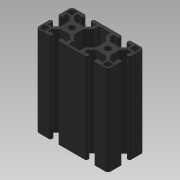
# Autodesk Inventor part: 40-4080-LITE-BLACK-FB
Saved by Autodesk Inventor 2013 (Build 170138000, 138)
## iProperties
Company: 80/20 Inc.
Created: 2014-04-23
Part Number: 40-4080-LITE-BLACK-FB
Material: Generic
Document SubType Name: Modeling
Designer: Ross Bowman
Density: 1 g/cm^3
Engineer: Ross Bowman
Catalog Web Link: 8020.net
Vendor: 80/20 Inc.
Material: 6105-T5 Aluminum
Author: Ross Bowman
Keywords: 80/20 , 8020 , T-Slot , Extrusion
Autodesk Inventor part; units mm, degrees
ref_plane "YZ Plane" through (0, 0, 0) normal (1, 0, 0) x (0, 1, 0)
ref_plane "XZ Plane" through (0, 0, 0) normal (0, 1, 0) x (-1, 0, 0)
ref_plane "XY Plane" through (0, 0, 0) normal (0, 0, 1) x (1, 0, 0)
sketch "Sketch1" plane through (0, 0, 0) normal (0, 0, 1) x (1, 0, 0)
  line L0 (31.935, -13.21) -> (31.935, -17.72)
  arc A0 (33.21, -11.94) -> (31.935, -13.21) centre (33.205, -13.21) ccw
  line L1 (37.72, -11.94) -> (33.21, -11.94)
  arc A1 (38.345, -12.57) -> (37.72, -11.94) centre (37.715, -12.57) ccw
  line L2 (38.345, -15.55) -> (38.345, -12.57)
  arc A2 (35.545, -18.35) -> (38.345, -15.55) centre (35.545, -15.55) ccw
  line L3 (32.565, -18.35) -> (35.545, -18.35)
  arc A3 (31.935, -17.72) -> (32.565, -18.35) centre (32.565, -17.72) ccw
  circle A4 centre (20, 0) radius 3.4
  line L4 (38.345, 12.57) -> (38.345, 15.55)
  arc A5 (37.72, 11.94) -> (38.345, 12.57) centre (37.715, 12.57) ccw
  line L5 (33.21, 11.94) -> (37.72, 11.94)
  arc A6 (31.935, 13.21) -> (33.21, 11.94) centre (33.205, 13.21) ccw
  line L6 (31.935, 17.72) -> (31.935, 13.21)
  arc A7 (32.565, 18.35) -> (31.935, 17.72) centre (32.565, 17.72) ccw
  line L7 (35.545, 18.35) -> (32.565, 18.35)
  arc A8 (38.345, 15.55) -> (35.545, 18.35) centre (35.545, 15.55) ccw
  line L8 (-38.345, -12.57) -> (-38.345, -15.55)
  arc A9 (-37.72, -11.94) -> (-38.345, -12.57) centre (-37.715, -12.57) ccw
  line L9 (-33.21, -11.94) -> (-37.72, -11.94)
  arc A10 (-31.935, -13.21) -> (-33.21, -11.94) centre (-33.205, -13.21) ccw
  line L10 (-31.935, -17.72) -> (-31.935, -13.21)
  arc A11 (-32.565, -18.35) -> (-31.935, -17.72) centre (-32.565, -17.72) ccw
  line L11 (-35.545, -18.35) -> (-32.565, -18.35)
  arc A12 (-38.345, -15.55) -> (-35.545, -18.35) centre (-35.545, -15.55) ccw
  line L12 (-10.9397, -6.7352) -> (-6.8324, -10.8426)
  arc A13 (-12.3289, -3.3756) -> (-10.9397, -6.7352) centre (-7.5789, -3.3786) ccw
  line L13 (-12.3247, 3.3825) -> (-12.3289, -3.3756)
  arc A14 (-10.9313, 6.7404) -> (-12.3247, 3.3825) centre (-7.5747, 3.3795) ccw
  line L14 (-6.8214, 10.8451) -> (-10.9313, 6.7404)
  arc A15 (-6.8214, 10.8451) -> (-6.4494, 11.7432) centre (-7.7194, 11.7432) ccw
  line L15 (-6.4494, 15.43) -> (-6.4494, 11.7432)
  arc A16 (-5.1787, 16.7) -> (-6.4494, 15.43) centre (-5.1794, 15.43) ccw
  line L16 (0, 16.6968) -> (-5.1787, 16.7)
  line L17 (5.1794, 16.7) -> (0, 16.6968)
  arc A17 (6.4494, 15.43) -> (5.1794, 16.7) centre (5.1794, 15.43) ccw
  line L18 (6.4494, 11.7432) -> (6.4494, 15.43)
  arc A18 (6.4494, 11.7432) -> (6.8214, 10.8451) centre (7.7194, 11.7432) ccw
  line L19 (10.9313, 6.7404) -> (6.8214, 10.8451)
  arc A19 (12.3247, 3.3825) -> (10.9313, 6.7404) centre (7.5747, 3.3795) ccw
  line L20 (12.3289, -3.3756) -> (12.3247, 3.3825)
  arc A20 (10.9376, -6.7373) -> (12.3289, -3.3756) centre (7.5789, -3.3786) ccw
  line L21 (6.8324, -10.8426) -> (10.9376, -6.7373)
  arc A21 (6.8324, -10.8426) -> (6.4604, -11.7406) centre (7.7304, -11.7406) ccw
  line L22 (6.4604, -16.4474) -> (6.4604, -11.7406)
  arc A22 (5.1904, -17.7174) -> (6.4604, -16.4474) centre (5.1904, -16.4474) ccw
  line L23 (-5.1904, -17.7174) -> (5.1904, -17.7174)
  arc A23 (-6.4604, -16.4474) -> (-5.1904, -17.7174) centre (-5.1904, -16.4474) ccw
  line L24 (-6.4604, -11.7406) -> (-6.4604, -16.4474)
  arc A24 (-6.4604, -11.7406) -> (-6.8324, -10.8426) centre (-7.7304, -11.7406) ccw
  circle A25 centre (-20, 0) radius 3.4
  line L25 (-37.72, 11.94) -> (-33.21, 11.94)
  arc A26 (-38.345, 12.57) -> (-37.72, 11.94) centre (-37.715, 12.57) ccw
  line L26 (-38.345, 15.55) -> (-38.345, 12.57)
  arc A27 (-35.545, 18.35) -> (-38.345, 15.55) centre (-35.545, 15.55) ccw
  line L27 (-32.565, 18.35) -> (-35.545, 18.35)
  arc A28 (-31.935, 17.72) -> (-32.565, 18.35) centre (-32.565, 17.72) ccw
  line L28 (-31.935, 13.21) -> (-31.935, 17.72)
  arc A29 (-33.21, 11.94) -> (-31.935, 13.21) centre (-33.205, 13.21) ccw
  arc A30 (-14.38, 20) -> (-15.94, 18.6069) centre (-14.38, 18.43) ccw
  line L29 (-15.94, 18.6069) -> (-15.94, 17.51)
  arc A31 (-15.94, 17.51) -> (-14.37, 15.94) centre (-14.37, 17.51) ccw
  line L30 (-14.37, 15.94) -> (-13.1517, 15.94)
  line L31 (-13.1517, 15.94) -> (-13.1517, 16.4117)
  line L32 (-13.1517, 16.4117) -> (-11.0437, 16.4117)
  arc A32 (-9.715, 15.1431) -> (-11.0437, 16.4117) centre (-10.985, 15.1431) ccw
  line L33 (-9.715, 15.1431) -> (-9.715, 12.8476)
  arc A33 (-9.9761, 12.2179) -> (-9.715, 12.8476) centre (-10.605, 12.8476) ccw
  line L34 (-9.9761, 12.2179) -> (-13.4586, 8.7397)
  arc A34 (-16.4245, 7.7) -> (-13.4586, 8.7397) centre (-16.4245, 12.45) ccw
  line L35 (-16.4245, 7.7) -> (-23.1872, 7.7)
  arc A35 (-26.7456, 9.087) -> (-23.1872, 7.7) centre (-23.3868, 12.4458) ccw
  line L36 (-26.7456, 9.087) -> (-30.0243, 12.3658)
  arc A36 (-30.285, 12.9951) -> (-30.0243, 12.3658) centre (-29.395, 12.9951) ccw
  line L37 (-30.285, 12.9951) -> (-30.285, 15.0869)
  arc A37 (-29.015, 16.3569) -> (-30.285, 15.0869) centre (-29.015, 15.0869) ccw
  line L38 (-29.015, 16.3569) -> (-26.8483, 16.3569)
  line L39 (-26.8483, 16.3569) -> (-26.8483, 15.8852)
  line L40 (-26.8483, 15.8852) -> (-25.63, 15.8852)
  arc A38 (-25.63, 15.8852) -> (-24.06, 17.4552) centre (-25.63, 17.4552) ccw
  line L41 (-24.06, 17.4552) -> (-24.06, 18.43)
  arc A39 (-24.06, 18.43) -> (-25.63, 20) centre (-25.63, 18.43) ccw
  line L42 (-25.63, 20) -> (-36.83, 20)
  arc A40 (-36.83, 20) -> (-40, 16.83) centre (-36.83, 16.83) ccw
  line L43 (-40, 16.83) -> (-40, 5.5719)
  arc A41 (-40, 5.5719) -> (-38.4311, 4.06) centre (-38.4311, 5.63) ccw
  line L44 (-38.4311, 4.06) -> (-37.51, 4.06)
  arc A42 (-37.51, 4.06) -> (-35.94, 5.63) centre (-37.51, 5.63) ccw
  line L45 (-35.94, 5.63) -> (-35.94, 6.6964)
  line L46 (-35.94, 6.6964) -> (-36.715, 6.6964)
  line L47 (-36.715, 6.6964) -> (-36.715, 9.02)
  arc A43 (-35.445, 10.29) -> (-36.715, 9.02) centre (-35.445, 9.02) ccw
  line L48 (-35.445, 10.29) -> (-33.1501, 10.29)
  arc A44 (-32.5208, 10.0293) -> (-33.1501, 10.29) centre (-33.1501, 9.4) ccw
  line L49 (-32.5208, 10.0293) -> (-29.0912, 6.5998)
  arc A45 (-27.7, 3.241) -> (-29.0912, 6.5998) centre (-32.45, 3.241) ccw
  line L50 (-27.7, 3.241) -> (-27.7, -3.241)
  arc A46 (-29.0912, -6.5998) -> (-27.7, -3.241) centre (-32.45, -3.241) ccw
  line L51 (-29.0912, -6.5998) -> (-32.5208, -10.0293)
  arc A47 (-33.1501, -10.29) -> (-32.5208, -10.0293) centre (-33.1501, -9.4) ccw
  line L52 (-33.1501, -10.29) -> (-35.445, -10.29)
  arc A48 (-36.715, -9.02) -> (-35.445, -10.29) centre (-35.445, -9.02) ccw
  line L53 (-36.715, -9.02) -> (-36.715, -6.6964)
  line L54 (-36.715, -6.6964) -> (-35.94, -6.6964)
  line L55 (-35.94, -6.6964) -> (-35.94, -5.63)
  arc A49 (-35.94, -5.63) -> (-37.51, -4.06) centre (-37.51, -5.63) ccw
  line L56 (-37.51, -4.06) -> (-38.4311, -4.06)
  arc A50 (-38.4311, -4.06) -> (-40, -5.5719) centre (-38.4311, -5.63) ccw
  line L57 (-40, -5.5719) -> (-40, -16.83)
  arc A51 (-40, -16.83) -> (-36.83, -20) centre (-36.83, -16.83) ccw
  line L58 (-36.83, -20) -> (-25.6944, -20)
  arc A52 (-25.6944, -20) -> (-24.06, -18.3656) centre (-25.6944, -18.3656) ccw
  line L59 (-24.06, -18.3656) -> (-24.06, -17.4474)
  arc A53 (-24.06, -17.4474) -> (-25.6944, -15.813) centre (-25.6944, -17.4474) ccw
  line L60 (-25.6944, -15.813) -> (-26.8283, -15.813)
  line L61 (-26.8283, -15.813) -> (-26.8283, -16.5584)
  line L62 (-26.8283, -16.5584) -> (-29.015, -16.5584)
  arc A54 (-30.285, -15.2884) -> (-29.015, -16.5584) centre (-29.015, -15.2884) ccw
  line L63 (-30.285, -15.2884) -> (-30.285, -12.8291)
  arc A55 (-30.0243, -12.1998) -> (-30.285, -12.8291) centre (-29.395, -12.8291) ccw
  line L64 (-30.0243, -12.1998) -> (-26.7392, -8.9146)
  arc A56 (-23.3804, -7.5234) -> (-26.7392, -8.9146) centre (-23.3804, -12.2734) ccw
  line L65 (-23.3804, -7.5234) -> (-16.6196, -7.5234)
  arc A57 (-13.2608, -8.9146) -> (-16.6196, -7.5234) centre (-16.6196, -12.2734) ccw
  line L66 (-13.2608, -8.9146) -> (-9.9757, -12.1998)
  arc A58 (-9.715, -12.8291) -> (-9.9757, -12.1998) centre (-10.605, -12.8291) ccw
  line L67 (-9.715, -12.8291) -> (-9.715, -15.3686)
  arc A59 (-11.0293, -16.5584) -> (-9.715, -15.3686) centre (-10.9825, -15.2892) ccw
  line L68 (-11.0293, -16.5584) -> (-13.1717, -16.5584)
  line L69 (-13.1717, -16.5584) -> (-13.1717, -15.813)
  line L70 (-13.1717, -15.813) -> (-14.3056, -15.813)
  arc A60 (-14.3056, -15.813) -> (-15.94, -17.4474) centre (-14.3056, -17.4474) ccw
  line L71 (-15.94, -17.4474) -> (-15.94, -18.3656)
  arc A61 (-15.94, -18.3656) -> (-14.3056, -20) centre (-14.3056, -18.3656) ccw
  line L72 (-14.3056, -20) -> (14.3056, -20)
  arc A62 (14.3056, -20) -> (15.94, -18.3656) centre (14.3056, -18.3656) ccw
  line L73 (15.94, -18.3656) -> (15.94, -17.4474)
  arc A63 (15.94, -17.4474) -> (14.3056, -15.813) centre (14.3056, -17.4474) ccw
  line L74 (14.3056, -15.813) -> (13.1717, -15.813)
  line L75 (13.1717, -15.813) -> (13.1717, -16.5584)
  line L76 (13.1717, -16.5584) -> (11.0293, -16.5584)
  arc A64 (9.715, -15.3686) -> (11.0293, -16.5584) centre (10.9825, -15.2892) ccw
  line L77 (9.715, -15.3686) -> (9.715, -12.8291)
  arc A65 (9.9757, -12.1998) -> (9.715, -12.8291) centre (10.605, -12.8291) ccw
  line L78 (9.9757, -12.1998) -> (13.2608, -8.9146)
  arc A66 (16.6196, -7.5234) -> (13.2608, -8.9146) centre (16.6196, -12.2734) ccw
  line L79 (16.6196, -7.5234) -> (23.3834, -7.5234)
  arc A67 (26.7392, -8.9146) -> (23.3834, -7.5234) centre (23.3804, -12.2734) ccw
  line L80 (26.7392, -8.9146) -> (30.0243, -12.1998)
  arc A68 (30.285, -12.8291) -> (30.0243, -12.1998) centre (29.395, -12.8291) ccw
  line L81 (30.285, -12.8291) -> (30.285, -15.2884)
  arc A69 (29.015, -16.5584) -> (30.285, -15.2884) centre (29.015, -15.2884) ccw
  line L82 (29.015, -16.5584) -> (26.907, -16.5584)
  line L83 (26.907, -16.5584) -> (26.907, -15.8852)
  line L84 (26.907, -15.8852) -> (25.63, -15.8852)
  arc A70 (25.63, -15.8852) -> (24.06, -17.4552) centre (25.63, -17.4552) ccw
  line L85 (24.06, -17.4552) -> (24.06, -18.4313)
  arc A71 (24.06, -18.4313) -> (25.6944, -20) centre (25.63, -18.4313) ccw
  line L86 (25.6944, -20) -> (36.83, -20)
  arc A72 (36.83, -20) -> (40, -16.83) centre (36.83, -16.83) ccw
  line L87 (40, -16.83) -> (40, -5.5696)
  arc A73 (40, -5.5696) -> (38.43, -3.9996) centre (38.43, -5.5696) ccw
  line L88 (38.43, -3.9996) -> (37.51, -3.9996)
  arc A74 (37.51, -3.9996) -> (35.94, -5.5696) centre (37.51, -5.5696) ccw
  line L89 (35.94, -5.5696) -> (35.94, -6.7799)
  line L90 (35.94, -6.7799) -> (36.5725, -6.7799)
  line L91 (36.5725, -6.7799) -> (36.5725, -9.1555)
  arc A75 (35.3025, -10.4255) -> (36.5725, -9.1555) centre (35.3025, -9.1555) ccw
  line L92 (35.3025, -10.4255) -> (33.0076, -10.4255)
  arc A76 (32.3778, -10.1644) -> (33.0076, -10.4255) centre (33.0076, -9.5355) ccw
  line L93 (32.3778, -10.1644) -> (29.0891, -6.8716)
  arc A77 (27.7, -3.515) -> (29.0891, -6.8716) centre (32.45, -3.515) ccw
  line L94 (27.7, -3.515) -> (27.7, 3.241)
  arc A78 (29.0912, 6.5998) -> (27.7, 3.241) centre (32.45, 3.241) ccw
  line L95 (29.0912, 6.5998) -> (32.5208, 10.0293)
  arc A79 (33.1501, 10.29) -> (32.5208, 10.0293) centre (33.1501, 9.4) ccw
  line L96 (33.1501, 10.29) -> (35.445, 10.29)
  arc A80 (36.715, 9.02) -> (35.445, 10.29) centre (35.445, 9.02) ccw
  line L97 (36.715, 9.02) -> (36.715, 6.6964)
  line L98 (36.715, 6.6964) -> (35.94, 6.6964)
  line L99 (35.94, 6.6964) -> (35.94, 5.63)
  arc A81 (35.94, 5.63) -> (37.51, 4.06) centre (37.51, 5.63) ccw
  line L100 (37.51, 4.06) -> (38.4311, 4.06)
  arc A82 (38.4311, 4.06) -> (40, 5.5719) centre (38.4311, 5.63) ccw
  line L101 (40, 5.5719) -> (40, 16.83)
  arc A83 (40, 16.83) -> (36.83, 20) centre (36.83, 16.83) ccw
  line L102 (36.83, 20) -> (25.63, 20)
  arc A84 (25.63, 20) -> (24.06, 18.43) centre (25.63, 18.43) ccw
  line L103 (24.06, 18.43) -> (24.06, 17.4552)
  arc A85 (24.06, 17.4552) -> (25.63, 15.8852) centre (25.63, 17.4552) ccw
  line L104 (25.63, 15.8852) -> (26.8483, 15.8852)
  line L105 (26.8483, 15.8852) -> (26.8483, 16.3569)
  line L106 (26.8483, 16.3569) -> (29.015, 16.3569)
  arc A86 (30.285, 15.0869) -> (29.015, 16.3569) centre (29.015, 15.0869) ccw
  line L107 (30.285, 15.0869) -> (30.285, 12.9951)
  arc A87 (30.0243, 12.3658) -> (30.285, 12.9951) centre (29.395, 12.9951) ccw
  line L108 (30.0243, 12.3658) -> (26.7456, 9.087)
  arc A88 (23.1872, 7.7) -> (26.7456, 9.087) centre (23.3868, 12.4458) ccw
  line L109 (23.1872, 7.7) -> (16.4312, 7.7)
  arc A89 (13.4586, 8.7397) -> (16.4312, 7.7) centre (16.4245, 12.45) ccw
  line L110 (13.4586, 8.7397) -> (9.9761, 12.2179)
  arc A90 (9.715, 12.8476) -> (9.9761, 12.2179) centre (10.605, 12.8476) ccw
  line L111 (9.715, 12.8476) -> (9.715, 15.1431)
  arc A91 (11.0437, 16.4117) -> (9.715, 15.1431) centre (10.985, 15.1431) ccw
  line L112 (11.0437, 16.4117) -> (13.1517, 16.4117)
  line L113 (13.1517, 16.4117) -> (13.1517, 15.94)
  line L114 (13.1517, 15.94) -> (14.37, 15.94)
  arc A92 (14.37, 15.94) -> (15.94, 17.51) centre (14.37, 17.51) ccw
  line L115 (15.94, 17.51) -> (15.94, 18.6069)
  arc A93 (15.94, 18.6069) -> (14.38, 20) centre (14.38, 18.43) ccw
  line L116 (14.38, 20) -> (-14.38, 20)
  point P0 (0, 0)
  constraints: 234 end point, 184 point on circle, 94 centre point
extrude "Extrusion1" add sketch "Sketch1" against normal blind 100
body "Solid1"
